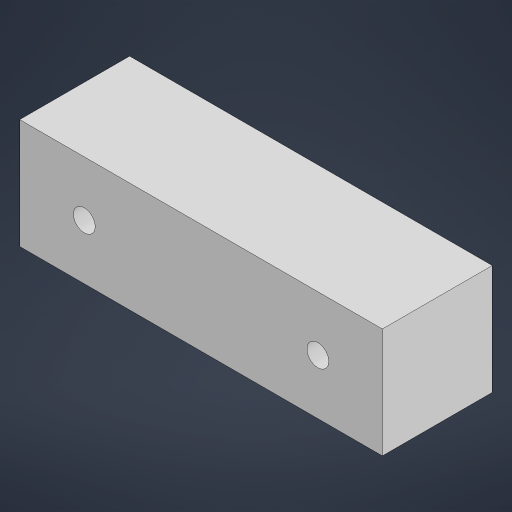
# Autodesk Inventor part: Tap_Zigu
Saved by Autodesk Inventor 2024.2 (Build 282272000, 272)
## iProperties
Created: 2024-01-22
Part Number: Tap_Zigu
Material: 一般
Document SubType Name: Modeling
Designer: Hanaoka
Density: 1 g/cm^3
Appearance: 既定
Author: Hanaoka
Autodesk Inventor part; units mm, degrees
ref_plane "YZ Plane" through (0, 0, 0) normal (1, 0, 0) x (0, 1, 0)
ref_plane "XZ Plane" through (0, 0, 0) normal (0, 1, 0) x (-1, 0, 0)
ref_plane "XY Plane" through (0, 0, 0) normal (0, 0, 1) x (1, 0, 0)
ref_plane "作業平面1" through (0, 0, 0) normal (0, 0, 1) x (1, 0, 0)
sketch "スケッチ1" plane through (0, 0, 0) normal (0, 0, 1) x (1, 0, 0)
  circle A0 centre (2.5, 2) radius 0.8 projected
  circle A1 centre (19.5, 2) radius 0.8 projected
  line L0 (0, 0) -> (22, 0) projected
  line L1 (22, 0) -> (22, 4) projected
  line L2 (0, 4) -> (22, 4) projected
  line L3 (0, 0) -> (0, 4) projected
  line L4 (24.2, 6) -> (-2.2, 6)
  line L5 (-2.2, 6) -> (-2.2, -2)
  line L6 (-2.2, -2) -> (24.2, -2)
  line L7 (24.2, -2) -> (24.2, 6)
  line L8 (24.2, 6) -> (-2.2, -2) construction
  line L9 (-2.2, 6) -> (24.2, -2) construction
  line L10 (22.2, 4) -> (-0.2, 4)
  line L11 (-0.2, 4) -> (-0.2, 0)
  line L12 (-0.2, 0) -> (22.2, 0)
  line L13 (22.2, 0) -> (22.2, 4)
  line L14 (22.2, 4) -> (-0.2, 0) construction
  line L15 (-0.2, 4) -> (22.2, 0) construction
  line L16 (11, 0) -> (11, 4) construction
  point P0 (11, 2)
  dimension "d0" = 0.2
  dimension "d1" = 0
  dimension "d2" = 2
  dimension "d3" = 2
  constraints: 26 end point, 7 midpoint, 4 parallel, 2 horizontal, 2 perpendicular
  measures "d0" distance between parallel lines of L11 L3
  measures "d1" distance between parallel lines of L12 L0
  measures "d2" distance between parallel lines of L5 L11
  measures "d3" distance between parallel lines of L4 L10
extrude "押し出し1" add sketch "スケッチ1" along normal blind 2 contours L3 L2 L1 L0 | L12 L11 L10 L3 | L1 L10 L13 L12 | L7 L6 L5 L4
sketch "スケッチ3" plane through (0, 0, 0) normal (0, 0, -1) x (-1, 0, 0)
  line L0 (-22.2, 4) -> (0.2, 4) projected
  line L1 (-22.2, 0) -> (-22.2, 4) projected
  line L2 (0.2, 0) -> (-22.2, 0) projected
  line L3 (0.2, 4) -> (0.2, 0) projected
  circle A0 centre (-2.5, 2) radius 0.8 projected
  circle A1 centre (-19.5, 2) radius 0.8 projected
  line L4 (-24.2, 6) -> (2.2, 6) projected
  line L5 (-24.2, -2) -> (-24.2, 6) projected
  line L6 (2.2, -2) -> (-24.2, -2) projected
  line L7 (2.2, 6) -> (2.2, -2) projected
  point P0 (0, 0)
extrude "押し出し2" add sketch "スケッチ3" along normal blind 6 contours L4 L7 L6 L5
equation "\"d3\" = d2"
